Autodesk Inventor part; units mm, degrees
(part 2 of 3)
  line L1003 (-158.1, -101.9) -> (-158.1, -108.1)
  line L1004 (-151.9, -108.1) -> (-151.9, -101.9)
  line L1005 (-151.9, -108.1) -> (-151.9, -111.9) construction
  line L1006 (-141.9, -108.1) -> (-141.9, -101.9)
  line L1007 (-148.1, -108.1) -> (-141.9, -108.1)
  line L1008 (-141.9, -111.9) -> (-148.1, -111.9)
  line L1009 (-141.9, -108.1) -> (-141.9, -111.9) construction
  line L1010 (-148.1, -101.9) -> (-148.1, -108.1)
  line L1011 (-151.9, -148.1) -> (-151.9, -151.9) construction
  line L1012 (-158.1, -148.1) -> (-151.9, -148.1)
  line L1013 (-141.9, -151.9) -> (-148.1, -151.9)
  line L1014 (-151.9, -141.9) -> (-158.1, -141.9)
  line L1015 (-158.1, -141.9) -> (-158.1, -148.1)
  line L1016 (-151.9, -148.1) -> (-151.9, -141.9)
  line L1017 (-148.1, -148.1) -> (-141.9, -148.1)
  line L1018 (-148.1, -141.9) -> (-148.1, -148.1)
  line L1019 (-141.9, -148.1) -> (-141.9, -141.9)
  line L1020 (-141.9, -148.1) -> (-141.9, -151.9) construction
  line L1021 (-141.9, -81.9) -> (-148.1, -81.9)
  line L1022 (-148.1, -81.9) -> (-148.1, -88.1)
  line L1023 (-148.1, -88.1) -> (-141.9, -88.1)
  line L1024 (-141.9, -88.1) -> (-141.9, -81.9)
  line L1025 (-151.9, -101.9) -> (-158.1, -101.9)
  line L1026 (-148.1, -98.1) -> (-141.9, -98.1)
  line L1027 (-141.9, -98.1) -> (-141.9, -101.9) construction
  line L1028 (-141.9, -91.9) -> (-148.1, -91.9)
  line L1029 (-148.1, -91.9) -> (-148.1, -98.1)
  line L1030 (-141.9, -98.1) -> (-141.9, -91.9)
  line L1031 (-141.9, -88.1) -> (-141.9, -91.9) construction
  line L1032 (-158.1, -98.1) -> (-151.9, -98.1)
  line L1033 (-151.9, -98.1) -> (-151.9, -101.9) construction
  line L1034 (-148.1, -178.1) -> (-141.9, -178.1)
  line L1035 (-148.1, -171.9) -> (-148.1, -178.1)
  line L1036 (-141.9, -178.1) -> (-141.9, -171.9)
  line L1037 (-151.9, -168.1) -> (-151.9, -171.9) construction
  line L1038 (-158.1, -168.1) -> (-151.9, -168.1)
  line L1039 (-151.9, -161.9) -> (-158.1, -161.9)
  line L1040 (-158.1, -161.9) -> (-158.1, -168.1)
  line L1041 (-151.9, -168.1) -> (-151.9, -161.9)
  line L1042 (-141.9, -171.9) -> (-148.1, -171.9)
  line L1043 (-148.1, -161.9) -> (-148.1, -168.1)
  line L1044 (-148.1, -168.1) -> (-141.9, -168.1)
  line L1045 (-141.9, -168.1) -> (-141.9, -171.9) construction
  line L1046 (-141.9, -161.9) -> (-148.1, -161.9)
  line L1047 (-141.9, -168.1) -> (-141.9, -161.9)
  line L1048 (-161.9, -78.1) -> (-161.9, -81.9) construction
  line L1049 (-171.9, -88.1) -> (-171.9, -91.9) construction
  line L1050 (-171.9, -98.1) -> (-171.9, -91.9)
  line L1051 (-178.1, -91.9) -> (-178.1, -98.1)
  line L1052 (-171.9, -91.9) -> (-178.1, -91.9)
  line L1053 (-171.9, -88.1) -> (-171.9, -81.9)
  line L1054 (-178.1, -88.1) -> (-171.9, -88.1)
  line L1055 (-178.1, -81.9) -> (-178.1, -88.1)
  line L1056 (-171.9, -81.9) -> (-178.1, -81.9)
  line L1057 (-171.9, -78.1) -> (-171.9, -81.9) construction
  line L1058 (-158.1, -68.1) -> (-151.9, -68.1)
  line L1059 (-151.9, -68.1) -> (-151.9, -71.9) construction
  line L1060 (-141.9, -68.1) -> (-141.9, -71.9) construction
  line L1061 (-158.1, -78.1) -> (-151.9, -78.1)
  line L1062 (-158.1, -71.9) -> (-158.1, -78.1)
  line L1063 (-151.9, -78.1) -> (-151.9, -71.9)
  line L1064 (-141.9, -71.9) -> (-148.1, -71.9)
  line L1065 (-148.1, -71.9) -> (-148.1, -78.1)
  line L1066 (-148.1, -78.1) -> (-141.9, -78.1)
  line L1067 (-141.9, -78.1) -> (-141.9, -71.9)
  line L1068 (-141.9, -78.1) -> (-141.9, -81.9) construction
  line L1069 (-151.9, -71.9) -> (-158.1, -71.9)
  line L1070 (-161.9, -78.1) -> (-161.9, -71.9)
  line L1071 (-168.1, -71.9) -> (-168.1, -78.1)
  line L1072 (-168.1, -78.1) -> (-161.9, -78.1)
  line L1073 (-161.9, -71.9) -> (-168.1, -71.9)
  line L1074 (-168.1, -68.1) -> (-161.9, -68.1)
  line L1075 (-161.9, -68.1) -> (-161.9, -61.9)
  line L1076 (-168.1, -61.9) -> (-168.1, -68.1)
  line L1077 (-161.9, -61.9) -> (-168.1, -61.9)
  line L1078 (-171.9, -68.1) -> (-171.9, -71.9) construction
  line L1079 (-171.9, -68.1) -> (-171.9, -61.9)
  line L1080 (-161.9, -68.1) -> (-161.9, -71.9) construction
  line L1081 (-148.1, -31.9) -> (-148.1, -38.1)
  line L1082 (-141.9, -31.9) -> (-148.1, -31.9)
  line L1083 (-148.1, -38.1) -> (-141.9, -38.1)
  line L1084 (-141.9, -38.1) -> (-141.9, -31.9)
  line L1085 (-141.9, -38.1) -> (-141.9, -41.9) construction
  line L1086 (-148.1, -118.1) -> (-141.9, -118.1)
  line L1087 (-141.9, -118.1) -> (-141.9, -111.9)
  line L1088 (-148.1, -111.9) -> (-148.1, -118.1)
  line L1089 (-141.9, -121.9) -> (-148.1, -121.9)
  line L1090 (-151.9, -111.9) -> (-158.1, -111.9)
  line L1091 (-151.9, -118.1) -> (-151.9, -111.9)
  line L1092 (-158.1, -111.9) -> (-158.1, -118.1)
  line L1093 (-158.1, -118.1) -> (-151.9, -118.1)
  line L1094 (-151.9, -121.9) -> (-158.1, -121.9)
  line L1095 (-151.9, -118.1) -> (-151.9, -121.9) construction
  line L1096 (-141.9, -118.1) -> (-141.9, -121.9) construction
  line L1097 (-158.1, -121.9) -> (-158.1, -128.1)
  line L1098 (-151.9, -128.1) -> (-151.9, -121.9)
  line L1099 (-148.1, -121.9) -> (-148.1, -128.1)
  line L1100 (-141.9, -128.1) -> (-141.9, -121.9)
  line L1101 (-148.1, -128.1) -> (-141.9, -128.1)
  line L1102 (-151.9, -171.9) -> (-158.1, -171.9)
  line L1103 (-158.1, -171.9) -> (-158.1, -178.1)
  line L1104 (-158.1, -178.1) -> (-151.9, -178.1)
  line L1105 (-151.9, -178.1) -> (-151.9, -171.9)
  line L1106 (-141.9, -128.1) -> (-141.9, -131.9) construction
  line L1107 (-141.9, -131.9) -> (-148.1, -131.9)
  line L1108 (-148.1, -131.9) -> (-148.1, -138.1)
  line L1109 (-148.1, -138.1) -> (-141.9, -138.1)
  line L1110 (-141.9, -138.1) -> (-141.9, -131.9)
  line L1111 (-141.9, -141.9) -> (-148.1, -141.9)
  line L1112 (-141.9, -138.1) -> (-141.9, -141.9) construction
  line L1113 (-158.1, -128.1) -> (-151.9, -128.1)
  line L1114 (-151.9, -131.9) -> (-158.1, -131.9)
  line L1115 (-151.9, -128.1) -> (-151.9, -131.9) construction
  line L1116 (-158.1, -138.1) -> (-151.9, -138.1)
  line L1117 (-158.1, -131.9) -> (-158.1, -138.1)
  line L1118 (-151.9, -138.1) -> (-151.9, -141.9) construction
  line L1119 (-151.9, -138.1) -> (-151.9, -131.9)
  line L1120 (-151.9, -151.9) -> (-158.1, -151.9)
  line L1121 (-148.1, -158.1) -> (-141.9, -158.1)
  line L1122 (-148.1, -151.9) -> (-148.1, -158.1)
  line L1123 (-141.9, -158.1) -> (-141.9, -151.9)
  line L1124 (-141.9, -158.1) -> (-141.9, -161.9) construction
  line L1125 (-158.1, -151.9) -> (-158.1, -158.1)
  line L1126 (-158.1, -158.1) -> (-151.9, -158.1)
  line L1127 (-151.9, -158.1) -> (-151.9, -161.9) construction
  line L1128 (-151.9, -158.1) -> (-151.9, -151.9)
  line L1129 (-161.9, -28.1) -> (-161.9, -31.9) construction
  line L1130 (-161.9, -28.1) -> (-161.9, -21.9)
  line L1131 (-161.9, -31.9) -> (-168.1, -31.9)
  line L1132 (-161.9, -21.9) -> (-168.1, -21.9)
  line L1133 (-168.1, -28.1) -> (-161.9, -28.1)
  line L1134 (-168.1, -21.9) -> (-168.1, -28.1)
  line L1135 (-171.9, -28.1) -> (-171.9, -31.9) construction
  line L1136 (-171.9, -21.9) -> (-168.1, -21.9) construction
  line L1137 (-171.9, -28.1) -> (-171.9, -21.9)
  line L1138 (-178.1, -28.1) -> (-171.9, -28.1)
  line L1139 (-171.9, -21.9) -> (-178.1, -21.9)
  line L1140 (-178.1, -21.9) -> (-178.1, -28.1)
  line L1141 (-151.9, -48.1) -> (-151.9, -51.9) construction
  line L1142 (-151.9, -41.9) -> (-158.1, -41.9)
  line L1143 (-158.1, -41.9) -> (-158.1, -48.1)
  line L1144 (-151.9, -48.1) -> (-151.9, -41.9)
  line L1145 (-151.9, -38.1) -> (-151.9, -41.9) construction
  line L1146 (-158.1, -48.1) -> (-151.9, -48.1)
  line L1147 (-178.1, -48.1) -> (-171.9, -48.1)
  line L1148 (-161.9, -48.1) -> (-161.9, -41.9)
  line L1149 (-168.1, -41.9) -> (-168.1, -48.1)
  line L1150 (-178.1, -41.9) -> (-178.1, -48.1)
  line L1151 (-171.9, -48.1) -> (-171.9, -41.9)
  line L1152 (-171.9, -51.9) -> (-178.1, -51.9)
  line L1153 (-171.9, -48.1) -> (-171.9, -51.9) construction
  line L1154 (-168.1, -48.1) -> (-161.9, -48.1)
  line L1155 (-171.9, -58.1) -> (-171.9, -51.9)
  line L1156 (-161.9, -51.9) -> (-168.1, -51.9)
  line L1157 (-161.9, -48.1) -> (-161.9, -51.9) construction
  line L1158 (-178.1, -58.1) -> (-171.9, -58.1)
  line L1159 (-178.1, -51.9) -> (-178.1, -58.1)
  line L1160 (-168.1, -51.9) -> (-168.1, -58.1)
  line L1161 (-168.1, -58.1) -> (-161.9, -58.1)
  line L1162 (-161.9, -58.1) -> (-161.9, -51.9)
  line L1163 (-161.9, -58.1) -> (-161.9, -61.9) construction
  line L1164 (-171.9, -58.1) -> (-171.9, -61.9) construction
  line L1165 (-168.1, -38.1) -> (-161.9, -38.1)
  line L1166 (-168.1, -31.9) -> (-168.1, -38.1)
  line L1167 (-161.9, -38.1) -> (-161.9, -31.9)
  line L1168 (-161.9, -41.9) -> (-168.1, -41.9)
  line L1169 (-161.9, -38.1) -> (-161.9, -41.9) construction
  line L1170 (-171.9, -38.1) -> (-171.9, -31.9)
  line L1171 (-171.9, -31.9) -> (-178.1, -31.9)
  line L1172 (-178.1, -38.1) -> (-171.9, -38.1)
  line L1173 (-178.1, -31.9) -> (-178.1, -38.1)
  line L1174 (-171.9, -38.1) -> (-171.9, -41.9) construction
  line L1175 (-171.9, -41.9) -> (-178.1, -41.9)
  line L1176 (-178.1, -98.1) -> (-171.9, -98.1)
  line L1177 (-168.1, -98.1) -> (-161.9, -98.1)
  line L1178 (-171.9, -98.1) -> (-171.9, -101.9) construction
  line L1179 (-161.9, -98.1) -> (-161.9, -101.9) construction
  line L1180 (-161.9, -101.9) -> (-168.1, -101.9)
  line L1181 (-171.9, -101.9) -> (-178.1, -101.9)
  line L1182 (-178.1, -101.9) -> (-178.1, -108.1)
  line L1183 (-171.9, -108.1) -> (-171.9, -101.9)
  line L1184 (-168.1, -101.9) -> (-168.1, -108.1)
  line L1185 (-161.9, -108.1) -> (-161.9, -101.9)
  line L1186 (-171.9, -61.9) -> (-178.1, -61.9)
  line L1187 (-178.1, -61.9) -> (-178.1, -68.1)
  line L1188 (-178.1, -68.1) -> (-171.9, -68.1)
  line L1189 (-171.9, -78.1) -> (-171.9, -71.9)
  line L1190 (-171.9, -71.9) -> (-178.1, -71.9)
  line L1191 (-178.1, -78.1) -> (-171.9, -78.1)
  line L1192 (-178.1, -71.9) -> (-178.1, -78.1)
  line L1193 (-161.9, -158.1) -> (-161.9, -161.9) construction
  line L1194 (-161.9, -161.9) -> (-168.1, -161.9)
  line L1195 (-171.9, -158.1) -> (-171.9, -151.9)
  line L1196 (-161.9, -168.1) -> (-161.9, -161.9)
  line L1197 (-168.1, -168.1) -> (-161.9, -168.1)
  line L1198 (-171.9, -151.9) -> (-178.1, -151.9)
  line L1199 (-178.1, -151.9) -> (-178.1, -158.1)
  line L1200 (-178.1, -158.1) -> (-171.9, -158.1)
  line L1201 (-171.9, -158.1) -> (-171.9, -161.9) construction
  line L1202 (-168.1, -161.9) -> (-168.1, -168.1)
  line L1203 (-171.9, -161.9) -> (-178.1, -161.9)
  line L1204 (-171.9, -168.1) -> (-171.9, -161.9)
  line L1205 (-178.1, -161.9) -> (-178.1, -168.1)
  line L1206 (-178.1, -168.1) -> (-171.9, -168.1)
  line L1207 (-161.9, -138.1) -> (-161.9, -131.9)
  line L1208 (-168.1, -131.9) -> (-168.1, -138.1)
  line L1209 (-161.9, -131.9) -> (-168.1, -131.9)
  line L1210 (-161.9, -128.1) -> (-161.9, -131.9) construction
  line L1211 (-168.1, -128.1) -> (-161.9, -128.1)
  line L1212 (-171.9, -138.1) -> (-171.9, -131.9)
  line L1213 (-161.9, -128.1) -> (-161.9, -121.9)
  line L1214 (-178.1, -138.1) -> (-171.9, -138.1)
  line L1215 (-178.1, -131.9) -> (-178.1, -138.1)
  line L1216 (-171.9, -131.9) -> (-178.1, -131.9)
  line L1217 (-171.9, -128.1) -> (-171.9, -131.9) construction
  line L1218 (-168.1, -121.9) -> (-168.1, -128.1)
  line L1219 (-161.9, -121.9) -> (-168.1, -121.9)
  line L1220 (-171.9, -128.1) -> (-171.9, -121.9)
  line L1221 (-178.1, -128.1) -> (-171.9, -128.1)
  line L1222 (-178.1, -121.9) -> (-178.1, -128.1)
  line L1223 (-161.9, -118.1) -> (-161.9, -121.9) construction
  line L1224 (-168.1, -118.1) -> (-161.9, -118.1)
  line L1225 (-161.9, -118.1) -> (-161.9, -111.9)
  line L1226 (-168.1, -111.9) -> (-168.1, -118.1)
  line L1227 (-161.9, -111.9) -> (-168.1, -111.9)
  line L1228 (-171.9, -118.1) -> (-171.9, -121.9) construction
  line L1229 (-171.9, -121.9) -> (-178.1, -121.9)
  line L1230 (-161.9, -108.1) -> (-161.9, -111.9) construction
  line L1231 (-171.9, -118.1) -> (-171.9, -111.9)
  line L1232 (-168.1, -108.1) -> (-161.9, -108.1)
  line L1233 (-178.1, -118.1) -> (-171.9, -118.1)
  line L1234 (-178.1, -111.9) -> (-178.1, -118.1)
  line L1235 (-171.9, -111.9) -> (-178.1, -111.9)
  line L1236 (-171.9, -108.1) -> (-171.9, -111.9) construction
  line L1237 (-178.1, -108.1) -> (-171.9, -108.1)
  line L1238 (-171.9, -148.1) -> (-171.9, -151.9) construction
  line L1239 (-168.1, -151.9) -> (-168.1, -158.1)
  line L1240 (-161.9, -158.1) -> (-161.9, -151.9)
  line L1241 (-161.9, -151.9) -> (-168.1, -151.9)
  line L1242 (-161.9, -148.1) -> (-161.9, -151.9) construction
  line L1243 (-168.1, -158.1) -> (-161.9, -158.1)
  line L1244 (-161.9, -168.1) -> (-161.9, -171.9) construction
  line L1245 (-168.1, -178.1) -> (-161.9, -178.1)
  line L1246 (-161.9, -171.9) -> (-168.1, -171.9)
  line L1247 (-168.1, -171.9) -> (-168.1, -178.1)
  line L1248 (-171.9, -168.1) -> (-171.9, -171.9) construction
  line L1249 (-171.9, -178.1) -> (-171.9, -171.9)
  line L1250 (-171.9, -171.9) -> (-178.1, -171.9)
  line L1251 (-178.1, -178.1) -> (-171.9, -178.1)
  line L1252 (-178.1, -171.9) -> (-178.1, -178.1)
  line L1253 (-161.9, -178.1) -> (-161.9, -171.9)
  line L1254 (-171.9, -141.9) -> (-178.1, -141.9)
  line L1255 (-178.1, -141.9) -> (-178.1, -148.1)
  line L1256 (-178.1, -148.1) -> (-171.9, -148.1)
  line L1257 (-171.9, -148.1) -> (-171.9, -141.9)
  line L1258 (-168.1, -138.1) -> (-161.9, -138.1)
  line L1259 (-171.9, -138.1) -> (-171.9, -141.9) construction
  line L1260 (-161.9, -138.1) -> (-161.9, -141.9) construction
  line L1261 (-161.9, -141.9) -> (-168.1, -141.9)
  line L1262 (-168.1, -141.9) -> (-168.1, -148.1)
  line L1263 (-161.9, -148.1) -> (-161.9, -141.9)
  line L1264 (-168.1, -148.1) -> (-161.9, -148.1)
  line L1265 (-151.9, -81.9) -> (-158.1, -81.9)
  line L1266 (-158.1, -88.1) -> (-151.9, -88.1)
  line L1267 (-151.9, -88.1) -> (-151.9, -81.9)
  line L1268 (-158.1, -81.9) -> (-158.1, -88.1)
  line L1269 (-151.9, -78.1) -> (-151.9, -81.9) construction
  line L1270 (-151.9, -91.9) -> (-158.1, -91.9)
  line L1271 (-168.1, -91.9) -> (-168.1, -98.1)
  line L1272 (-168.1, -81.9) -> (-168.1, -88.1)
  line L1273 (-168.1, -88.1) -> (-161.9, -88.1)
  line L1274 (-161.9, -81.9) -> (-168.1, -81.9)
  line L1275 (-161.9, -91.9) -> (-168.1, -91.9)
  line L1276 (-161.9, -88.1) -> (-161.9, -91.9) construction
  line L1277 (-161.9, -98.1) -> (-161.9, -91.9)
  line L1278 (-158.1, -91.9) -> (-158.1, -98.1)
  line L1279 (-151.9, -88.1) -> (-151.9, -91.9) construction
  line L1280 (-151.9, -98.1) -> (-151.9, -91.9)
  line L1281 (-161.9, -88.1) -> (-161.9, -81.9)
  line L1282 (-21.9, -178.1) -> (-10, -178.1) construction
  line L1283 (-178.1, -21.9) -> (-178.1, -10) construction
  line L1284 (-178.1, -21.9) -> (-190, -21.9) construction
  line L1285 (-178.1, -178.1) -> (-190, -178.1) construction
  line L1286 (-178.1, -178.1) -> (-178.1, -190) construction
  line L1287 (-10, -21.9) -> (-10, -178.1)
  line L1288 (-10, -178.1) -> (0, -178.1)
  line L1289 (0, -178.1) -> (0, -200)
  line L1290 (0, -200) -> (-21.9, -200)
  line L1291 (-21.9, -200) -> (-21.9, -190)
  line L1292 (-21.9, -190) -> (-178.1, -190)
  line L1293 (-178.1, -190) -> (-178.1, -200)
  line L1294 (-178.1, -200) -> (-200, -200)
  line L1295 (-200, -200) -> (-200, -178.1)
  line L1296 (-200, -178.1) -> (-190, -178.1)
  line L1297 (-190, -21.9) -> (-190, -178.1)
  line L1298 (-190, -21.9) -> (-200, -21.9)
  line L1299 (-200, -21.9) -> (-200, 0)
  line L1300 (-200, 0) -> (-178.1, 0)
  line L1301 (-178.1, 0) -> (-178.1, -10)
  line L1302 (-178.1, -10) -> (-21.9, -10)
  line L1303 (-21.9, -10) -> (-21.9, 0)
  line L1304 (-21.9, 0) -> (0, 0)
  line L1305 (0, 0) -> (0, -21.9)
  line L1306 (0, -21.9) -> (-10, -21.9)
  dimension "d10" = 3.8
  dimension "d11" = 6.2
  dimension "d51" = 11.9
  dimension "d84" = 21.9
  constraints: 2614 end point, 635 equal length, 512 parallel, 378 point on line, 301 perpendicular, 269 horizontal, 151 vertical, 2 collinear, 1 coincident
  measures "d10" distance of L2.end L4.start
  measures "d11" distance of L0.start L0.end
  measures "d51" distance of L0.start L24.end
  measures "d84" distance of L1304.end L1305.end
extrude "Extrusion3" add sketch "Skizze1" along normal blind 2
sketch "Skizze2" plane through (0, 2, 0) normal (0, 1, 0) x (1, 0, 0)
  line L0 (20.9, 20.9) -> (29.1, 20.9)
  line L1 (29.1, 20.9) -> (29.1, 29.1)
  line L2 (29.1, 29.1) -> (20.9, 29.1)
  line L3 (20.9, 29.1) -> (20.9, 20.9)
  line L4 (20.9, 30.9) -> (29.1, 30.9)
  line L5 (29.1, 30.9) -> (29.1, 39.1)
  line L6 (29.1, 39.1) -> (20.9, 39.1)
  line L7 (20.9, 39.1) -> (20.9, 30.9)
  line L8 (20.9, 29.1) -> (20.9, 30.9) construction
  line L9 (20.9, 40.9) -> (29.1, 40.9)
  line L10 (29.1, 40.9) -> (29.1, 49.1)
  line L11 (29.1, 49.1) -> (20.9, 49.1)
  line L12 (20.9, 49.1) -> (20.9, 40.9)
  line L13 (20.9, 50.9) -> (29.1, 50.9)
  line L14 (29.1, 50.9) -> (29.1, 59.1)
  line L15 (29.1, 59.1) -> (20.9, 59.1)
  line L16 (20.9, 59.1) -> (20.9, 50.9)
  line L17 (20.9, 49.1) -> (20.9, 50.9) construction
  line L18 (20.9, 39.1) -> (20.9, 40.9) construction
  line L19 (21.9, 21.9) -> (21.9, 20.9) construction
  line L20 (28.1, 21.9) -> (21.9, 21.9) construction
  line L21 (21.9, 21.9) -> (20.9, 21.9) construction
  line L22 (20.9, 60.9) -> (29.1, 60.9)
  line L23 (29.1, 60.9) -> (29.1, 69.1)
  line L24 (29.1, 69.1) -> (20.9, 69.1)
  line L25 (20.9, 69.1) -> (20.9, 60.9)
  line L26 (20.9, 70.9) -> (29.1, 70.9)
  line L27 (29.1, 70.9) -> (29.1, 79.1)
  line L28 (29.1, 79.1) -> (20.9, 79.1)
  line L29 (20.9, 79.1) -> (20.9, 70.9)
  line L30 (20.9, 69.1) -> (20.9, 70.9) construction
  line L31 (20.9, 80.9) -> (29.1, 80.9)
  line L32 (29.1, 80.9) -> (29.1, 89.1)
  line L33 (29.1, 89.1) -> (20.9, 89.1)
  line L34 (20.9, 89.1) -> (20.9, 80.9)
  line L35 (20.9, 90.9) -> (29.1, 90.9)
  line L36 (29.1, 90.9) -> (29.1, 99.1)
  line L37 (29.1, 99.1) -> (20.9, 99.1)
  line L38 (20.9, 99.1) -> (20.9, 90.9)
  line L39 (20.9, 89.1) -> (20.9, 90.9) construction
  line L40 (20.9, 79.1) -> (20.9, 80.9) construction
  line L41 (20.9, 60.9) -> (20.9, 59.1) construction
  line L42 (20.9, 100.9) -> (29.1, 100.9)
  line L43 (29.1, 100.9) -> (29.1, 109.1)
  line L44 (29.1, 109.1) -> (20.9, 109.1)
  line L45 (20.9, 109.1) -> (20.9, 100.9)
  line L46 (20.9, 110.9) -> (29.1, 110.9)
  line L47 (29.1, 110.9) -> (29.1, 119.1)
  line L48 (29.1, 119.1) -> (20.9, 119.1)
  line L49 (20.9, 119.1) -> (20.9, 110.9)
  line L50 (20.9, 109.1) -> (20.9, 110.9) construction
  line L51 (20.9, 120.9) -> (29.1, 120.9)
  line L52 (29.1, 120.9) -> (29.1, 129.1)
  line L53 (29.1, 129.1) -> (20.9, 129.1)
  line L54 (20.9, 129.1) -> (20.9, 120.9)
  line L55 (20.9, 130.9) -> (29.1, 130.9)
  line L56 (29.1, 130.9) -> (29.1, 139.1)
  line L57 (29.1, 139.1) -> (20.9, 139.1)
  line L58 (20.9, 139.1) -> (20.9, 130.9)
  line L59 (20.9, 129.1) -> (20.9, 130.9) construction
  line L60 (20.9, 119.1) -> (20.9, 120.9) construction
  line L61 (29.1, 159.1) -> (20.9, 159.1)
  line L62 (20.9, 159.1) -> (20.9, 160.9) construction
  line L63 (20.9, 160.9) -> (29.1, 160.9)
  line L64 (29.1, 160.9) -> (29.1, 169.1)
  line L65 (29.1, 169.1) -> (20.9, 169.1)
  line L66 (20.9, 170.9) -> (29.1, 170.9)
  line L67 (20.9, 169.1) -> (20.9, 170.9) construction
  line L68 (29.1, 170.9) -> (29.1, 179.1)
  line L69 (29.1, 179.1) -> (20.9, 179.1)
  line L70 (20.9, 179.1) -> (20.9, 170.9)
  line L71 (20.9, 169.1) -> (20.9, 160.9)
  line L72 (20.9, 140.9) -> (29.1, 140.9)
  line L73 (29.1, 140.9) -> (29.1, 149.1)
  line L74 (29.1, 149.1) -> (20.9, 149.1)
  line L75 (20.9, 149.1) -> (20.9, 140.9)
  line L76 (29.1, 150.9) -> (29.1, 159.1)
  line L77 (20.9, 159.1) -> (20.9, 150.9)
  line L78 (20.9, 150.9) -> (29.1, 150.9)
  line L79 (20.9, 149.1) -> (20.9, 150.9) construction
  line L80 (20.9, 140.9) -> (20.9, 139.1) construction
  line L81 (20.9, 99.1) -> (20.9, 100.9) construction
  line L82 (30.9, 20.9) -> (39.1, 20.9)
  line L83 (39.1, 20.9) -> (39.1, 29.1)
  line L84 (39.1, 29.1) -> (30.9, 29.1)
  line L85 (30.9, 29.1) -> (30.9, 20.9)
  line L86 (30.9, 30.9) -> (39.1, 30.9)
  line L87 (39.1, 30.9) -> (39.1, 39.1)
  line L88 (39.1, 39.1) -> (30.9, 39.1)
  line L89 (30.9, 39.1) -> (30.9, 30.9)
  line L90 (30.9, 29.1) -> (30.9, 30.9) construction
  line L91 (30.9, 40.9) -> (39.1, 40.9)
  line L92 (39.1, 40.9) -> (39.1, 49.1)
  line L93 (39.1, 49.1) -> (30.9, 49.1)
  line L94 (30.9, 49.1) -> (30.9, 40.9)
  line L95 (30.9, 50.9) -> (39.1, 50.9)
  line L96 (39.1, 50.9) -> (39.1, 59.1)
  line L97 (39.1, 59.1) -> (30.9, 59.1)
  line L98 (30.9, 59.1) -> (30.9, 50.9)
  line L99 (30.9, 49.1) -> (30.9, 50.9) construction
  line L100 (30.9, 39.1) -> (30.9, 40.9) construction
  line L101 (39.1, 79.1) -> (30.9, 79.1)
  line L102 (30.9, 79.1) -> (30.9, 80.9) construction
  line L103 (30.9, 80.9) -> (39.1, 80.9)
  line L104 (39.1, 80.9) -> (39.1, 89.1)
  line L105 (39.1, 89.1) -> (30.9, 89.1)
  line L106 (30.9, 90.9) -> (39.1, 90.9)
  line L107 (30.9, 89.1) -> (30.9, 90.9) construction
  line L108 (39.1, 90.9) -> (39.1, 99.1)
  line L109 (39.1, 99.1) -> (30.9, 99.1)
  line L110 (30.9, 99.1) -> (30.9, 90.9)
  line L111 (30.9, 89.1) -> (30.9, 80.9)
  line L112 (30.9, 60.9) -> (39.1, 60.9)
  line L113 (39.1, 60.9) -> (39.1, 69.1)
  line L114 (39.1, 69.1) -> (30.9, 69.1)
  line L115 (30.9, 69.1) -> (30.9, 60.9)
  line L116 (39.1, 70.9) -> (39.1, 79.1)
  line L117 (30.9, 79.1) -> (30.9, 70.9)
  line L118 (30.9, 70.9) -> (39.1, 70.9)
  line L119 (30.9, 69.1) -> (30.9, 70.9) construction
  line L120 (30.9, 60.9) -> (30.9, 59.1) construction
  line L121 (39.1, 110.9) -> (39.1, 119.1)
  line L122 (30.9, 119.1) -> (30.9, 110.9)
  line L123 (39.1, 119.1) -> (30.9, 119.1)
  line L124 (30.9, 119.1) -> (30.9, 120.9) construction
  line L125 (30.9, 120.9) -> (39.1, 120.9)
  line L126 (39.1, 120.9) -> (39.1, 129.1)
  line L127 (30.9, 129.1) -> (30.9, 120.9)
  line L128 (39.1, 129.1) -> (30.9, 129.1)
  line L129 (30.9, 130.9) -> (39.1, 130.9)
  line L130 (30.9, 129.1) -> (30.9, 130.9) construction
  line L131 (39.1, 130.9) -> (39.1, 139.1)
  line L132 (30.9, 139.1) -> (30.9, 130.9)
  line L133 (39.1, 139.1) -> (30.9, 139.1)
  line L134 (30.9, 140.9) -> (30.9, 139.1) construction
  line L135 (30.9, 140.9) -> (39.1, 140.9)
  line L136 (30.9, 149.1) -> (30.9, 140.9)
  line L137 (39.1, 140.9) -> (39.1, 149.1)
  line L138 (39.1, 149.1) -> (30.9, 149.1)
  line L139 (30.9, 149.1) -> (30.9, 150.9) construction
  line L140 (30.9, 150.9) -> (39.1, 150.9)
  line L141 (39.1, 159.1) -> (30.9, 159.1)
  line L142 (39.1, 150.9) -> (39.1, 159.1)
  line L143 (30.9, 159.1) -> (30.9, 150.9)
  line L144 (30.9, 110.9) -> (39.1, 110.9)
  line L145 (30.9, 109.1) -> (30.9, 110.9) construction
  line L146 (39.1, 109.1) -> (30.9, 109.1)
  line L147 (30.9, 109.1) -> (30.9, 100.9)
  line L148 (30.9, 100.9) -> (39.1, 100.9)
  line L149 (39.1, 100.9) -> (39.1, 109.1)
  line L150 (30.9, 159.1) -> (30.9, 160.9) construction
  line L151 (39.1, 160.9) -> (39.1, 169.1)
  line L152 (39.1, 169.1) -> (30.9, 169.1)
  line L153 (30.9, 169.1) -> (30.9, 160.9)
  line L154 (30.9, 170.9) -> (39.1, 170.9)
  line L155 (30.9, 169.1) -> (30.9, 170.9) construction
  line L156 (39.1, 170.9) -> (39.1, 179.1)
  line L157 (39.1, 179.1) -> (30.9, 179.1)
  line L158 (30.9, 179.1) -> (30.9, 170.9)
  line L159 (30.9, 160.9) -> (39.1, 160.9)
  line L160 (30.9, 99.1) -> (30.9, 100.9) construction
  line L161 (29.1, 20.9) -> (30.9, 20.9) construction
  line L162 (40.9, 20.9) -> (49.1, 20.9)
  line L163 (49.1, 20.9) -> (49.1, 29.1)
  line L164 (49.1, 29.1) -> (40.9, 29.1)
  line L165 (40.9, 29.1) -> (40.9, 20.9)
  line L166 (40.9, 30.9) -> (49.1, 30.9)
  line L167 (49.1, 30.9) -> (49.1, 39.1)
  line L168 (49.1, 39.1) -> (40.9, 39.1)
  line L169 (40.9, 39.1) -> (40.9, 30.9)
  line L170 (40.9, 29.1) -> (40.9, 30.9) construction
  line L171 (40.9, 40.9) -> (49.1, 40.9)
  line L172 (49.1, 40.9) -> (49.1, 49.1)
  line L173 (49.1, 49.1) -> (40.9, 49.1)
  line L174 (40.9, 49.1) -> (40.9, 40.9)
  line L175 (40.9, 50.9) -> (49.1, 50.9)
  line L176 (49.1, 50.9) -> (49.1, 59.1)
  line L177 (49.1, 59.1) -> (40.9, 59.1)
  line L178 (40.9, 59.1) -> (40.9, 50.9)
  line L179 (40.9, 49.1) -> (40.9, 50.9) construction
  line L180 (40.9, 39.1) -> (40.9, 40.9) construction
  line L181 (49.1, 79.1) -> (40.9, 79.1)
  line L182 (40.9, 79.1) -> (40.9, 80.9) construction
  line L183 (40.9, 80.9) -> (49.1, 80.9)
  line L184 (49.1, 80.9) -> (49.1, 89.1)
  line L185 (49.1, 89.1) -> (40.9, 89.1)
  line L186 (40.9, 90.9) -> (49.1, 90.9)
  line L187 (40.9, 89.1) -> (40.9, 90.9) construction
  line L188 (49.1, 90.9) -> (49.1, 99.1)
  line L189 (49.1, 99.1) -> (40.9, 99.1)
  line L190 (40.9, 99.1) -> (40.9, 90.9)
  line L191 (40.9, 89.1) -> (40.9, 80.9)
  line L192 (40.9, 60.9) -> (49.1, 60.9)
  line L193 (49.1, 60.9) -> (49.1, 69.1)
  line L194 (49.1, 69.1) -> (40.9, 69.1)
  line L195 (40.9, 69.1) -> (40.9, 60.9)
  line L196 (49.1, 70.9) -> (49.1, 79.1)
  line L197 (40.9, 79.1) -> (40.9, 70.9)
  line L198 (40.9, 70.9) -> (49.1, 70.9)
  line L199 (40.9, 69.1) -> (40.9, 70.9) construction
  line L200 (40.9, 60.9) -> (40.9, 59.1) construction
  line L201 (49.1, 110.9) -> (49.1, 119.1)
  line L202 (40.9, 119.1) -> (40.9, 110.9)
  line L203 (49.1, 119.1) -> (40.9, 119.1)
  line L204 (40.9, 119.1) -> (40.9, 120.9) construction
  line L205 (40.9, 120.9) -> (49.1, 120.9)
  line L206 (49.1, 120.9) -> (49.1, 129.1)
  line L207 (40.9, 129.1) -> (40.9, 120.9)
  line L208 (49.1, 129.1) -> (40.9, 129.1)
  line L209 (40.9, 130.9) -> (49.1, 130.9)
  line L210 (40.9, 129.1) -> (40.9, 130.9) construction
  line L211 (49.1, 130.9) -> (49.1, 139.1)
  line L212 (40.9, 139.1) -> (40.9, 130.9)
  line L213 (49.1, 139.1) -> (40.9, 139.1)
  line L214 (40.9, 140.9) -> (40.9, 139.1) construction
  line L215 (40.9, 140.9) -> (49.1, 140.9)
  line L216 (40.9, 149.1) -> (40.9, 140.9)
  line L217 (49.1, 140.9) -> (49.1, 149.1)
  line L218 (49.1, 149.1) -> (40.9, 149.1)
  line L219 (40.9, 149.1) -> (40.9, 150.9) construction
  line L220 (40.9, 150.9) -> (49.1, 150.9)
  line L221 (49.1, 159.1) -> (40.9, 159.1)
  line L222 (49.1, 150.9) -> (49.1, 159.1)
  line L223 (40.9, 159.1) -> (40.9, 150.9)
  line L224 (40.9, 110.9) -> (49.1, 110.9)
  line L225 (40.9, 109.1) -> (40.9, 110.9) construction
  line L226 (49.1, 109.1) -> (40.9, 109.1)
  line L227 (40.9, 109.1) -> (40.9, 100.9)
  line L228 (40.9, 100.9) -> (49.1, 100.9)
  line L229 (49.1, 100.9) -> (49.1, 109.1)
  line L230 (40.9, 159.1) -> (40.9, 160.9) construction
  line L231 (49.1, 160.9) -> (49.1, 169.1)
  line L232 (49.1, 169.1) -> (40.9, 169.1)
  line L233 (40.9, 169.1) -> (40.9, 160.9)
  line L234 (40.9, 170.9) -> (49.1, 170.9)
  line L235 (40.9, 169.1) -> (40.9, 170.9) construction
  line L236 (49.1, 170.9) -> (49.1, 179.1)
  line L237 (49.1, 179.1) -> (40.9, 179.1)
  line L238 (40.9, 179.1) -> (40.9, 170.9)
  line L239 (40.9, 160.9) -> (49.1, 160.9)
  line L240 (40.9, 99.1) -> (40.9, 100.9) construction
  line L241 (50.9, 20.9) -> (59.1, 20.9)
  line L242 (59.1, 20.9) -> (59.1, 29.1)
  line L243 (59.1, 29.1) -> (50.9, 29.1)
  line L244 (50.9, 29.1) -> (50.9, 20.9)
  line L245 (50.9, 30.9) -> (59.1, 30.9)
  line L246 (59.1, 30.9) -> (59.1, 39.1)
  line L247 (59.1, 39.1) -> (50.9, 39.1)
  line L248 (50.9, 39.1) -> (50.9, 30.9)
  line L249 (50.9, 29.1) -> (50.9, 30.9) construction
  line L250 (50.9, 39.1) -> (50.9, 40.9) construction
  line L251 (50.9, 40.9) -> (59.1, 40.9)
  line L252 (59.1, 40.9) -> (59.1, 49.1)
  line L253 (50.9, 49.1) -> (50.9, 40.9)
  line L254 (59.1, 49.1) -> (50.9, 49.1)
  line L255 (50.9, 49.1) -> (50.9, 50.9) construction
  line L256 (50.9, 50.9) -> (59.1, 50.9)
  line L257 (59.1, 50.9) -> (59.1, 59.1)
  line L258 (59.1, 59.1) -> (50.9, 59.1)
  line L259 (50.9, 60.9) -> (59.1, 60.9)
  line L260 (50.9, 60.9) -> (50.9, 59.1) construction
  line L261 (50.9, 59.1) -> (50.9, 50.9)
  line L262 (59.1, 89.1) -> (50.9, 89.1)
  line L263 (50.9, 90.9) -> (59.1, 90.9)
  line L264 (50.9, 89.1) -> (50.9, 90.9) construction
  line L265 (59.1, 90.9) -> (59.1, 99.1)
  line L266 (59.1, 99.1) -> (50.9, 99.1)
  line L267 (50.9, 99.1) -> (50.9, 90.9)
  line L268 (50.9, 99.1) -> (50.9, 100.9) construction
  line L269 (59.1, 109.1) -> (50.9, 109.1)
  line L270 (50.9, 109.1) -> (50.9, 100.9)
  line L271 (59.1, 100.9) -> (59.1, 109.1)
  line L272 (50.9, 110.9) -> (59.1, 110.9)
  line L273 (50.9, 109.1) -> (50.9, 110.9) construction
  line L274 (50.9, 119.1) -> (50.9, 110.9)
  line L275 (59.1, 110.9) -> (59.1, 119.1)
  line L276 (50.9, 100.9) -> (59.1, 100.9)
  line L277 (59.1, 119.1) -> (50.9, 119.1)
  line L278 (50.9, 119.1) -> (50.9, 120.9) construction
  line L279 (50.9, 120.9) -> (59.1, 120.9)
  line L280 (59.1, 120.9) -> (59.1, 129.1)
  line L281 (50.9, 129.1) -> (50.9, 120.9)
  line L282 (59.1, 139.1) -> (50.9, 139.1)
  line L283 (50.9, 140.9) -> (50.9, 139.1) construction
  line L284 (50.9, 130.9) -> (59.1, 130.9)
  line L285 (50.9, 139.1) -> (50.9, 130.9)
  line L286 (59.1, 129.1) -> (50.9, 129.1)
  line L287 (50.9, 129.1) -> (50.9, 130.9) construction
  line L288 (59.1, 130.9) -> (59.1, 139.1)
  line L289 (59.1, 160.9) -> (59.1, 169.1)
  line L290 (50.9, 169.1) -> (50.9, 160.9)
  line L291 (59.1, 169.1) -> (50.9, 169.1)
  line L292 (50.9, 169.1) -> (50.9, 170.9) construction
  line L293 (50.9, 170.9) -> (59.1, 170.9)
  line L294 (50.9, 179.1) -> (50.9, 170.9)
  line L295 (59.1, 170.9) -> (59.1, 179.1)
  line L296 (59.1, 179.1) -> (50.9, 179.1)
  line L297 (59.1, 149.1) -> (50.9, 149.1)
  line L298 (59.1, 140.9) -> (59.1, 149.1)
  line L299 (50.9, 150.9) -> (59.1, 150.9)
  line L300 (50.9, 149.1) -> (50.9, 150.9) construction
  line L301 (59.1, 150.9) -> (59.1, 159.1)
  line L302 (59.1, 159.1) -> (50.9, 159.1)
  line L303 (50.9, 159.1) -> (50.9, 150.9)
  line L304 (50.9, 160.9) -> (59.1, 160.9)
  line L305 (50.9, 159.1) -> (50.9, 160.9) construction
  line L306 (50.9, 149.1) -> (50.9, 140.9)
  line L307 (50.9, 140.9) -> (59.1, 140.9)
  line L308 (59.1, 60.9) -> (59.1, 69.1)
  line L309 (50.9, 69.1) -> (50.9, 60.9)
  line L310 (59.1, 69.1) -> (50.9, 69.1)
  line L311 (50.9, 69.1) -> (50.9, 70.9) construction
  line L312 (50.9, 70.9) -> (59.1, 70.9)
  line L313 (59.1, 70.9) -> (59.1, 79.1)
  line L314 (50.9, 79.1) -> (50.9, 70.9)
  line L315 (59.1, 79.1) -> (50.9, 79.1)
  line L316 (50.9, 79.1) -> (50.9, 80.9) construction
  line L317 (59.1, 80.9) -> (59.1, 89.1)
  line L318 (50.9, 89.1) -> (50.9, 80.9)
  line L319 (50.9, 80.9) -> (59.1, 80.9)
  line L320 (49.1, 20.9) -> (50.9, 20.9) construction
  line L321 (39.1, 20.9) -> (40.9, 20.9) construction
  line L322 (60.9, 20.9) -> (69.1, 20.9)
  line L323 (69.1, 20.9) -> (69.1, 29.1)
  line L324 (69.1, 29.1) -> (60.9, 29.1)
  line L325 (60.9, 29.1) -> (60.9, 20.9)
  line L326 (60.9, 30.9) -> (69.1, 30.9)
  line L327 (69.1, 30.9) -> (69.1, 39.1)
  line L328 (69.1, 39.1) -> (60.9, 39.1)
  line L329 (60.9, 39.1) -> (60.9, 30.9)
  line L330 (60.9, 29.1) -> (60.9, 30.9) construction
  line L331 (60.9, 40.9) -> (69.1, 40.9)
  line L332 (69.1, 40.9) -> (69.1, 49.1)
  line L333 (69.1, 49.1) -> (60.9, 49.1)
  line L334 (60.9, 49.1) -> (60.9, 40.9)
  line L335 (60.9, 50.9) -> (69.1, 50.9)
  line L336 (69.1, 50.9) -> (69.1, 59.1)
  line L337 (69.1, 59.1) -> (60.9, 59.1)
  line L338 (60.9, 59.1) -> (60.9, 50.9)
  line L339 (60.9, 49.1) -> (60.9, 50.9) construction
  line L340 (60.9, 39.1) -> (60.9, 40.9) construction
  line L341 (69.1, 79.1) -> (60.9, 79.1)
  line L342 (60.9, 79.1) -> (60.9, 80.9) construction
  line L343 (60.9, 80.9) -> (69.1, 80.9)
  line L344 (69.1, 80.9) -> (69.1, 89.1)
  line L345 (69.1, 89.1) -> (60.9, 89.1)
  line L346 (60.9, 90.9) -> (69.1, 90.9)
  line L347 (60.9, 89.1) -> (60.9, 90.9) construction
  line L348 (69.1, 90.9) -> (69.1, 99.1)
  line L349 (69.1, 99.1) -> (60.9, 99.1)
  line L350 (60.9, 99.1) -> (60.9, 90.9)
  line L351 (60.9, 89.1) -> (60.9, 80.9)
  line L352 (60.9, 60.9) -> (69.1, 60.9)
  line L353 (69.1, 60.9) -> (69.1, 69.1)
  line L354 (69.1, 69.1) -> (60.9, 69.1)
  line L355 (60.9, 69.1) -> (60.9, 60.9)
  line L356 (69.1, 70.9) -> (69.1, 79.1)
  line L357 (60.9, 79.1) -> (60.9, 70.9)
  line L358 (60.9, 70.9) -> (69.1, 70.9)
  line L359 (60.9, 69.1) -> (60.9, 70.9) construction
  line L360 (60.9, 60.9) -> (60.9, 59.1) construction
  line L361 (69.1, 110.9) -> (69.1, 119.1)
  line L362 (60.9, 119.1) -> (60.9, 110.9)
  line L363 (69.1, 119.1) -> (60.9, 119.1)
  line L364 (60.9, 119.1) -> (60.9, 120.9) construction
  line L365 (60.9, 120.9) -> (69.1, 120.9)
  line L366 (69.1, 120.9) -> (69.1, 129.1)
  line L367 (60.9, 129.1) -> (60.9, 120.9)
  line L368 (69.1, 129.1) -> (60.9, 129.1)
  line L369 (60.9, 130.9) -> (69.1, 130.9)
  line L370 (60.9, 129.1) -> (60.9, 130.9) construction
  line L371 (69.1, 130.9) -> (69.1, 139.1)
  line L372 (60.9, 139.1) -> (60.9, 130.9)
  line L373 (69.1, 139.1) -> (60.9, 139.1)
  line L374 (60.9, 140.9) -> (60.9, 139.1) construction
  line L375 (60.9, 140.9) -> (69.1, 140.9)
  line L376 (60.9, 149.1) -> (60.9, 140.9)
  line L377 (69.1, 140.9) -> (69.1, 149.1)
  line L378 (69.1, 149.1) -> (60.9, 149.1)
  line L379 (60.9, 149.1) -> (60.9, 150.9) construction
  line L380 (60.9, 150.9) -> (69.1, 150.9)
  line L381 (69.1, 159.1) -> (60.9, 159.1)
  line L382 (69.1, 150.9) -> (69.1, 159.1)
  line L383 (60.9, 159.1) -> (60.9, 150.9)
  line L384 (60.9, 110.9) -> (69.1, 110.9)
  line L385 (60.9, 109.1) -> (60.9, 110.9) construction
  line L386 (69.1, 109.1) -> (60.9, 109.1)
  line L387 (60.9, 109.1) -> (60.9, 100.9)
  line L388 (60.9, 100.9) -> (69.1, 100.9)
  line L389 (69.1, 100.9) -> (69.1, 109.1)
  line L390 (60.9, 159.1) -> (60.9, 160.9) construction
  line L391 (69.1, 160.9) -> (69.1, 169.1)
  line L392 (69.1, 169.1) -> (60.9, 169.1)
  line L393 (60.9, 169.1) -> (60.9, 160.9)
  line L394 (60.9, 170.9) -> (69.1, 170.9)
  line L395 (60.9, 169.1) -> (60.9, 170.9) construction
  line L396 (69.1, 170.9) -> (69.1, 179.1)
  line L397 (69.1, 179.1) -> (60.9, 179.1)
  line L398 (60.9, 179.1) -> (60.9, 170.9)
  line L399 (60.9, 160.9) -> (69.1, 160.9)
  line L400 (60.9, 99.1) -> (60.9, 100.9) construction
  line L401 (70.9, 20.9) -> (79.1, 20.9)
  line L402 (79.1, 20.9) -> (79.1, 29.1)
  line L403 (79.1, 29.1) -> (70.9, 29.1)
  line L404 (70.9, 29.1) -> (70.9, 20.9)
  line L405 (70.9, 30.9) -> (79.1, 30.9)
  line L406 (79.1, 30.9) -> (79.1, 39.1)
  line L407 (79.1, 39.1) -> (70.9, 39.1)
  line L408 (70.9, 39.1) -> (70.9, 30.9)
  line L409 (70.9, 29.1) -> (70.9, 30.9) construction
  line L410 (70.9, 39.1) -> (70.9, 40.9) construction
  line L411 (70.9, 40.9) -> (79.1, 40.9)
  line L412 (79.1, 40.9) -> (79.1, 49.1)
  line L413 (70.9, 49.1) -> (70.9, 40.9)
  line L414 (79.1, 49.1) -> (70.9, 49.1)
  line L415 (70.9, 49.1) -> (70.9, 50.9) construction
  line L416 (70.9, 50.9) -> (79.1, 50.9)
  line L417 (79.1, 50.9) -> (79.1, 59.1)
  line L418 (79.1, 59.1) -> (70.9, 59.1)
  line L419 (70.9, 60.9) -> (79.1, 60.9)
  line L420 (70.9, 60.9) -> (70.9, 59.1) construction
  line L421 (70.9, 59.1) -> (70.9, 50.9)
  line L422 (79.1, 89.1) -> (70.9, 89.1)
  line L423 (70.9, 90.9) -> (79.1, 90.9)
  line L424 (70.9, 89.1) -> (70.9, 90.9) construction
  line L425 (79.1, 90.9) -> (79.1, 99.1)
  line L426 (79.1, 99.1) -> (70.9, 99.1)
  line L427 (70.9, 99.1) -> (70.9, 90.9)
  line L428 (70.9, 99.1) -> (70.9, 100.9) construction
  line L429 (79.1, 109.1) -> (70.9, 109.1)
  line L430 (70.9, 109.1) -> (70.9, 100.9)
  line L431 (79.1, 100.9) -> (79.1, 109.1)
  line L432 (70.9, 110.9) -> (79.1, 110.9)
  line L433 (70.9, 109.1) -> (70.9, 110.9) construction
  line L434 (70.9, 119.1) -> (70.9, 110.9)
  line L435 (79.1, 110.9) -> (79.1, 119.1)
  line L436 (70.9, 100.9) -> (79.1, 100.9)
  line L437 (79.1, 119.1) -> (70.9, 119.1)
  line L438 (70.9, 119.1) -> (70.9, 120.9) construction
  line L439 (70.9, 120.9) -> (79.1, 120.9)
  line L440 (79.1, 120.9) -> (79.1, 129.1)
  line L441 (70.9, 129.1) -> (70.9, 120.9)
  line L442 (79.1, 139.1) -> (70.9, 139.1)
  line L443 (70.9, 140.9) -> (70.9, 139.1) construction
  line L444 (70.9, 130.9) -> (79.1, 130.9)
  line L445 (70.9, 139.1) -> (70.9, 130.9)
  line L446 (79.1, 129.1) -> (70.9, 129.1)
  line L447 (70.9, 129.1) -> (70.9, 130.9) construction
  line L448 (79.1, 130.9) -> (79.1, 139.1)
  line L449 (79.1, 160.9) -> (79.1, 169.1)
  line L450 (70.9, 169.1) -> (70.9, 160.9)
  line L451 (79.1, 169.1) -> (70.9, 169.1)
  line L452 (70.9, 169.1) -> (70.9, 170.9) construction
  line L453 (70.9, 170.9) -> (79.1, 170.9)
  line L454 (70.9, 179.1) -> (70.9, 170.9)
  line L455 (79.1, 170.9) -> (79.1, 179.1)
  line L456 (79.1, 179.1) -> (70.9, 179.1)
  line L457 (79.1, 149.1) -> (70.9, 149.1)
  line L458 (79.1, 140.9) -> (79.1, 149.1)
  line L459 (70.9, 150.9) -> (79.1, 150.9)
  line L460 (70.9, 149.1) -> (70.9, 150.9) construction
  line L461 (79.1, 150.9) -> (79.1, 159.1)
  line L462 (79.1, 159.1) -> (70.9, 159.1)
  line L463 (70.9, 159.1) -> (70.9, 150.9)
  line L464 (70.9, 160.9) -> (79.1, 160.9)
  line L465 (70.9, 159.1) -> (70.9, 160.9) construction
  line L466 (70.9, 149.1) -> (70.9, 140.9)
  line L467 (70.9, 140.9) -> (79.1, 140.9)
  line L468 (79.1, 60.9) -> (79.1, 69.1)
  line L469 (70.9, 69.1) -> (70.9, 60.9)
  line L470 (79.1, 69.1) -> (70.9, 69.1)
  line L471 (70.9, 69.1) -> (70.9, 70.9) construction
  line L472 (70.9, 70.9) -> (79.1, 70.9)
  line L473 (79.1, 70.9) -> (79.1, 79.1)
  line L474 (70.9, 79.1) -> (70.9, 70.9)
  line L475 (79.1, 79.1) -> (70.9, 79.1)
  line L476 (70.9, 79.1) -> (70.9, 80.9) construction
  line L477 (79.1, 80.9) -> (79.1, 89.1)
  line L478 (70.9, 89.1) -> (70.9, 80.9)
  line L479 (70.9, 80.9) -> (79.1, 80.9)
  line L480 (69.1, 20.9) -> (70.9, 20.9) construction
  line L481 (80.9, 20.9) -> (89.1, 20.9)
  line L482 (89.1, 20.9) -> (89.1, 29.1)
  line L483 (89.1, 29.1) -> (80.9, 29.1)
  line L484 (80.9, 29.1) -> (80.9, 20.9)
  line L485 (90.9, 20.9) -> (99.1, 20.9)
  line L486 (99.1, 20.9) -> (99.1, 29.1)
  line L487 (90.9, 29.1) -> (90.9, 20.9)
  line L488 (89.1, 20.9) -> (90.9, 20.9) construction
  line L489 (89.1, 89.1) -> (80.9, 89.1)
  line L490 (80.9, 90.9) -> (89.1, 90.9)
  line L491 (80.9, 89.1) -> (80.9, 90.9) construction
  line L492 (89.1, 90.9) -> (89.1, 99.1)
  line L493 (99.1, 90.9) -> (99.1, 99.1)
  line L494 (90.9, 90.9) -> (99.1, 90.9)
  line L495 (99.1, 89.1) -> (90.9, 89.1)
  line L496 (90.9, 99.1) -> (90.9, 90.9)
  line L497 (90.9, 89.1) -> (90.9, 90.9) construction
  line L498 (89.1, 99.1) -> (80.9, 99.1)
  line L499 (80.9, 100.9) -> (89.1, 100.9)
  line L500 (80.9, 99.1) -> (80.9, 100.9) construction
  line L501 (80.9, 99.1) -> (80.9, 90.9)
  line L502 (89.1, 59.1) -> (80.9, 59.1)
  line L503 (99.1, 59.1) -> (90.9, 59.1)
  line L504 (90.9, 60.9) -> (90.9, 59.1) construction
  line L505 (90.9, 60.9) -> (99.1, 60.9)
  line L506 (99.1, 60.9) -> (99.1, 69.1)
  line L507 (80.9, 60.9) -> (80.9, 59.1) construction
  line L508 (80.9, 60.9) -> (89.1, 60.9)
  line L509 (90.9, 69.1) -> (90.9, 60.9)
  line L510 (89.1, 60.9) -> (89.1, 69.1)
  line L511 (80.9, 69.1) -> (80.9, 60.9)
  line L512 (89.1, 69.1) -> (80.9, 69.1)
  line L513 (80.9, 70.9) -> (89.1, 70.9)
  line L514 (80.9, 69.1) -> (80.9, 70.9) construction
  line L515 (80.9, 140.9) -> (89.1, 140.9)
  line L516 (80.9, 140.9) -> (80.9, 139.1) construction
  line L517 (90.9, 139.1) -> (90.9, 130.9)
  line L518 (89.1, 139.1) -> (80.9, 139.1)
  line L519 (89.1, 130.9) -> (89.1, 139.1)
  line L520 (90.9, 129.1) -> (90.9, 130.9) construction
  line L521 (80.9, 139.1) -> (80.9, 130.9)
  line L522 (80.9, 130.9) -> (89.1, 130.9)
  line L523 (80.9, 129.1) -> (80.9, 130.9) construction
  line L524 (89.1, 129.1) -> (80.9, 129.1)
  line L525 (90.9, 140.9) -> (90.9, 139.1) construction
  line L526 (90.9, 130.9) -> (99.1, 130.9)
  line L527 (99.1, 130.9) -> (99.1, 139.1)
  line L528 (80.9, 149.1) -> (80.9, 140.9)
  line L529 (99.1, 139.1) -> (90.9, 139.1)
  line L530 (89.1, 140.9) -> (89.1, 149.1)
  line L531 (90.9, 140.9) -> (99.1, 140.9)
  line L532 (90.9, 149.1) -> (90.9, 140.9)
  line L533 (99.1, 140.9) -> (99.1, 149.1)
  line L534 (80.9, 30.9) -> (89.1, 30.9)
  line L535 (89.1, 30.9) -> (89.1, 39.1)
  line L536 (89.1, 39.1) -> (80.9, 39.1)
  line L537 (80.9, 39.1) -> (80.9, 30.9)
  line L538 (80.9, 29.1) -> (80.9, 30.9) construction
  line L539 (90.9, 29.1) -> (90.9, 30.9) construction
  line L540 (80.9, 40.9) -> (89.1, 40.9)
  line L541 (80.9, 39.1) -> (80.9, 40.9) construction
  line L542 (99.1, 29.1) -> (90.9, 29.1)
  line L543 (90.9, 39.1) -> (90.9, 30.9)
  line L544 (90.9, 30.9) -> (99.1, 30.9)
  line L545 (90.9, 39.1) -> (90.9, 40.9) construction
  line L546 (99.1, 30.9) -> (99.1, 39.1)
  line L547 (99.1, 39.1) -> (90.9, 39.1)
  line L548 (90.9, 40.9) -> (99.1, 40.9)
  line L549 (89.1, 40.9) -> (89.1, 49.1)
  line L550 (89.1, 49.1) -> (80.9, 49.1)
  line L551 (80.9, 49.1) -> (80.9, 40.9)
  line L552 (80.9, 50.9) -> (89.1, 50.9)
  line L553 (89.1, 50.9) -> (89.1, 59.1)
  line L554 (80.9, 59.1) -> (80.9, 50.9)
  line L555 (80.9, 49.1) -> (80.9, 50.9) construction
  line L556 (90.9, 59.1) -> (90.9, 50.9)
  line L557 (99.1, 50.9) -> (99.1, 59.1)
  line L558 (90.9, 49.1) -> (90.9, 50.9) construction
  line L559 (90.9, 50.9) -> (99.1, 50.9)
  line L560 (99.1, 49.1) -> (90.9, 49.1)
  line L561 (90.9, 49.1) -> (90.9, 40.9)
  line L562 (99.1, 40.9) -> (99.1, 49.1)
  line L563 (99.1, 109.1) -> (90.9, 109.1)
  line L564 (90.9, 109.1) -> (90.9, 110.9) construction
  line L565 (90.9, 110.9) -> (99.1, 110.9)
  line L566 (99.1, 119.1) -> (90.9, 119.1)
  line L567 (90.9, 119.1) -> (90.9, 110.9)
  line L568 (90.9, 119.1) -> (90.9, 120.9) construction
  line L569 (90.9, 120.9) -> (99.1, 120.9)
  line L570 (99.1, 110.9) -> (99.1, 119.1)
  line L571 (89.1, 110.9) -> (89.1, 119.1)
  line L572 (80.9, 119.1) -> (80.9, 110.9)
  line L573 (89.1, 119.1) -> (80.9, 119.1)
  line L574 (80.9, 119.1) -> (80.9, 120.9) construction
  line L575 (80.9, 120.9) -> (89.1, 120.9)
  line L576 (89.1, 120.9) -> (89.1, 129.1)
  line L577 (80.9, 129.1) -> (80.9, 120.9)
  line L578 (90.9, 129.1) -> (90.9, 120.9)
  line L579 (99.1, 120.9) -> (99.1, 129.1)
  line L580 (99.1, 129.1) -> (90.9, 129.1)
  line L581 (89.1, 149.1) -> (80.9, 149.1)
  line L582 (80.9, 149.1) -> (80.9, 150.9) construction
  line L583 (80.9, 150.9) -> (89.1, 150.9)
  line L584 (89.1, 159.1) -> (80.9, 159.1)
  line L585 (89.1, 150.9) -> (89.1, 159.1)
  line L586 (80.9, 159.1) -> (80.9, 150.9)
  line L587 (80.9, 159.1) -> (80.9, 160.9) construction
  line L588 (80.9, 160.9) -> (89.1, 160.9)
  line L589 (90.9, 150.9) -> (99.1, 150.9)
  line L590 (90.9, 149.1) -> (90.9, 150.9) construction
  line L591 (90.9, 159.1) -> (90.9, 150.9)
  line L592 (90.9, 159.1) -> (90.9, 160.9) construction
  line L593 (99.1, 159.1) -> (90.9, 159.1)
  line L594 (99.1, 150.9) -> (99.1, 159.1)
  line L595 (90.9, 160.9) -> (99.1, 160.9)
  line L596 (99.1, 149.1) -> (90.9, 149.1)
  line L597 (90.9, 99.1) -> (90.9, 100.9) construction
  line L598 (89.1, 109.1) -> (80.9, 109.1)
  line L599 (80.9, 109.1) -> (80.9, 100.9)
  line L600 (80.9, 110.9) -> (89.1, 110.9)
  line L601 (80.9, 109.1) -> (80.9, 110.9) construction
  line L602 (89.1, 100.9) -> (89.1, 109.1)
  line L603 (99.1, 99.1) -> (90.9, 99.1)
  line L604 (90.9, 109.1) -> (90.9, 100.9)
  line L605 (99.1, 100.9) -> (99.1, 109.1)
  line L606 (90.9, 100.9) -> (99.1, 100.9)
  line L607 (89.1, 79.1) -> (80.9, 79.1)
  line L608 (80.9, 79.1) -> (80.9, 80.9) construction
  line L609 (80.9, 80.9) -> (89.1, 80.9)
  line L610 (89.1, 80.9) -> (89.1, 89.1)
  line L611 (80.9, 89.1) -> (80.9, 80.9)
  line L612 (89.1, 70.9) -> (89.1, 79.1)
  line L613 (80.9, 79.1) -> (80.9, 70.9)
  line L614 (99.1, 69.1) -> (90.9, 69.1)
  line L615 (90.9, 69.1) -> (90.9, 70.9) construction
  line L616 (90.9, 70.9) -> (99.1, 70.9)
  line L617 (99.1, 70.9) -> (99.1, 79.1)
  line L618 (90.9, 79.1) -> (90.9, 70.9)
  line L619 (99.1, 79.1) -> (90.9, 79.1)
  line L620 (90.9, 79.1) -> (90.9, 80.9) construction
  line L621 (90.9, 80.9) -> (99.1, 80.9)
  line L622 (90.9, 89.1) -> (90.9, 80.9)
  line L623 (99.1, 80.9) -> (99.1, 89.1)
  line L624 (89.1, 160.9) -> (89.1, 169.1)
  line L625 (89.1, 169.1) -> (80.9, 169.1)
  line L626 (80.9, 169.1) -> (80.9, 160.9)
  line L627 (80.9, 170.9) -> (89.1, 170.9)
  line L628 (80.9, 169.1) -> (80.9, 170.9) construction
  line L629 (89.1, 170.9) -> (89.1, 179.1)
  line L630 (89.1, 179.1) -> (80.9, 179.1)
  line L631 (80.9, 179.1) -> (80.9, 170.9)
  line L632 (99.1, 160.9) -> (99.1, 169.1)
  line L633 (90.9, 169.1) -> (90.9, 160.9)
  line L634 (99.1, 169.1) -> (90.9, 169.1)
  line L635 (90.9, 169.1) -> (90.9, 170.9) construction
  line L636 (90.9, 179.1) -> (90.9, 170.9)
  line L637 (99.1, 170.9) -> (99.1, 179.1)
  line L638 (99.1, 179.1) -> (90.9, 179.1)
  line L639 (90.9, 170.9) -> (99.1, 170.9)
  line L640 (79.1, 20.9) -> (80.9, 20.9) construction
  line L641 (59.1, 20.9) -> (60.9, 20.9) construction
  line L642 (100.9, 20.9) -> (109.1, 20.9)
  line L643 (109.1, 20.9) -> (109.1, 29.1)
  line L644 (109.1, 29.1) -> (100.9, 29.1)
  line L645 (100.9, 29.1) -> (100.9, 20.9)
  line L646 (100.9, 30.9) -> (109.1, 30.9)
  line L647 (109.1, 30.9) -> (109.1, 39.1)
  line L648 (109.1, 39.1) -> (100.9, 39.1)
  line L649 (100.9, 39.1) -> (100.9, 30.9)
  line L650 (100.9, 29.1) -> (100.9, 30.9) construction
  line L651 (100.9, 40.9) -> (109.1, 40.9)
  line L652 (109.1, 40.9) -> (109.1, 49.1)
  line L653 (109.1, 49.1) -> (100.9, 49.1)
  line L654 (100.9, 49.1) -> (100.9, 40.9)
  line L655 (100.9, 50.9) -> (109.1, 50.9)
  line L656 (109.1, 50.9) -> (109.1, 59.1)
  line L657 (109.1, 59.1) -> (100.9, 59.1)
  line L658 (100.9, 59.1) -> (100.9, 50.9)
  line L659 (100.9, 49.1) -> (100.9, 50.9) construction
  line L660 (100.9, 39.1) -> (100.9, 40.9) construction
  line L661 (109.1, 79.1) -> (100.9, 79.1)
  line L662 (100.9, 79.1) -> (100.9, 80.9) construction
  line L663 (100.9, 80.9) -> (109.1, 80.9)
  line L664 (109.1, 80.9) -> (109.1, 89.1)
  line L665 (109.1, 89.1) -> (100.9, 89.1)
  line L666 (100.9, 90.9) -> (109.1, 90.9)
  line L667 (100.9, 89.1) -> (100.9, 90.9) construction
  line L668 (109.1, 90.9) -> (109.1, 99.1)
  line L669 (109.1, 99.1) -> (100.9, 99.1)
  line L670 (100.9, 99.1) -> (100.9, 90.9)
  line L671 (100.9, 89.1) -> (100.9, 80.9)
  line L672 (100.9, 60.9) -> (109.1, 60.9)
  line L673 (109.1, 60.9) -> (109.1, 69.1)
  line L674 (109.1, 69.1) -> (100.9, 69.1)
  line L675 (100.9, 69.1) -> (100.9, 60.9)
  line L676 (109.1, 70.9) -> (109.1, 79.1)
  line L677 (100.9, 79.1) -> (100.9, 70.9)
  line L678 (100.9, 70.9) -> (109.1, 70.9)
  line L679 (100.9, 69.1) -> (100.9, 70.9) construction
  line L680 (100.9, 60.9) -> (100.9, 59.1) construction
  line L681 (109.1, 110.9) -> (109.1, 119.1)
  line L682 (100.9, 119.1) -> (100.9, 110.9)
  line L683 (109.1, 119.1) -> (100.9, 119.1)
  line L684 (100.9, 119.1) -> (100.9, 120.9) construction
  line L685 (100.9, 120.9) -> (109.1, 120.9)
  line L686 (109.1, 120.9) -> (109.1, 129.1)
  line L687 (100.9, 129.1) -> (100.9, 120.9)
  line L688 (109.1, 129.1) -> (100.9, 129.1)
  line L689 (100.9, 130.9) -> (109.1, 130.9)
  line L690 (100.9, 129.1) -> (100.9, 130.9) construction
  line L691 (109.1, 130.9) -> (109.1, 139.1)
  line L692 (100.9, 139.1) -> (100.9, 130.9)
  line L693 (109.1, 139.1) -> (100.9, 139.1)
  line L694 (100.9, 140.9) -> (100.9, 139.1) construction
  line L695 (100.9, 140.9) -> (109.1, 140.9)
  line L696 (100.9, 149.1) -> (100.9, 140.9)
  line L697 (109.1, 140.9) -> (109.1, 149.1)
  line L698 (109.1, 149.1) -> (100.9, 149.1)
  line L699 (100.9, 149.1) -> (100.9, 150.9) construction
  line L700 (100.9, 150.9) -> (109.1, 150.9)
  line L701 (109.1, 159.1) -> (100.9, 159.1)
  line L702 (109.1, 150.9) -> (109.1, 159.1)
  line L703 (100.9, 159.1) -> (100.9, 150.9)
  line L704 (100.9, 110.9) -> (109.1, 110.9)
  line L705 (100.9, 109.1) -> (100.9, 110.9) construction
  line L706 (109.1, 109.1) -> (100.9, 109.1)
  line L707 (100.9, 109.1) -> (100.9, 100.9)
  line L708 (100.9, 100.9) -> (109.1, 100.9)
  line L709 (109.1, 100.9) -> (109.1, 109.1)
  line L710 (100.9, 159.1) -> (100.9, 160.9) construction
  line L711 (109.1, 160.9) -> (109.1, 169.1)
  line L712 (109.1, 169.1) -> (100.9, 169.1)
  line L713 (100.9, 169.1) -> (100.9, 160.9)
  line L714 (100.9, 170.9) -> (109.1, 170.9)
  line L715 (100.9, 169.1) -> (100.9, 170.9) construction
  line L716 (109.1, 170.9) -> (109.1, 179.1)
  line L717 (109.1, 179.1) -> (100.9, 179.1)
  line L718 (100.9, 179.1) -> (100.9, 170.9)
  line L719 (100.9, 160.9) -> (109.1, 160.9)
  line L720 (100.9, 99.1) -> (100.9, 100.9) construction
  line L721 (110.9, 20.9) -> (119.1, 20.9)
  line L722 (119.1, 20.9) -> (119.1, 29.1)
  line L723 (119.1, 29.1) -> (110.9, 29.1)
  line L724 (110.9, 29.1) -> (110.9, 20.9)
  line L725 (110.9, 30.9) -> (119.1, 30.9)
  line L726 (119.1, 30.9) -> (119.1, 39.1)
  line L727 (119.1, 39.1) -> (110.9, 39.1)
  line L728 (110.9, 39.1) -> (110.9, 30.9)
  line L729 (110.9, 29.1) -> (110.9, 30.9) construction
  line L730 (110.9, 39.1) -> (110.9, 40.9) construction
  line L731 (110.9, 40.9) -> (119.1, 40.9)
  line L732 (119.1, 40.9) -> (119.1, 49.1)
  line L733 (110.9, 49.1) -> (110.9, 40.9)
  line L734 (119.1, 49.1) -> (110.9, 49.1)
  line L735 (110.9, 49.1) -> (110.9, 50.9) construction
  line L736 (110.9, 50.9) -> (119.1, 50.9)
  line L737 (119.1, 50.9) -> (119.1, 59.1)
  line L738 (119.1, 59.1) -> (110.9, 59.1)
  line L739 (110.9, 60.9) -> (119.1, 60.9)
  line L740 (110.9, 60.9) -> (110.9, 59.1) construction
  line L741 (110.9, 59.1) -> (110.9, 50.9)
  line L742 (119.1, 89.1) -> (110.9, 89.1)
  line L743 (110.9, 90.9) -> (119.1, 90.9)
  line L744 (110.9, 89.1) -> (110.9, 90.9) construction
  line L745 (119.1, 90.9) -> (119.1, 99.1)
  line L746 (119.1, 99.1) -> (110.9, 99.1)
  line L747 (110.9, 99.1) -> (110.9, 90.9)
  line L748 (110.9, 99.1) -> (110.9, 100.9) construction
  line L749 (119.1, 109.1) -> (110.9, 109.1)
  line L750 (110.9, 109.1) -> (110.9, 100.9)
  line L751 (119.1, 100.9) -> (119.1, 109.1)
  line L752 (110.9, 110.9) -> (119.1, 110.9)
  line L753 (110.9, 109.1) -> (110.9, 110.9) construction
  line L754 (110.9, 119.1) -> (110.9, 110.9)